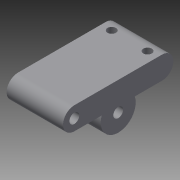
# Autodesk Inventor part: armv2
Saved by Autodesk Inventor 2015 (Build 190159000, 159)
## iProperties
Created: 2015-02-01
Part Number: armv2
Material: Generic
Document SubType Name: Modeling
Designer: Jumziey
Density: 1 g/cm^3
Appearance: Default
Author: Jumziey
Autodesk Inventor part; units mm, degrees
ref_plane "XZ Plane" through (0, 0, 0) normal (0, 1, 0) x (-1, 0, 0)
ref_plane "XY Plane" through (0, 0, 0) normal (0, 0, 1) x (1, 0, 0)
sketch "Sketch1" plane through (0, 0, 0) normal (1, 0, 0) x (0, 1, 0)
  circle A0 centre (0, 0) radius 1.75
  arc A1 (0, 4) -> (0, -4) centre (0, 0) ccw
  line L0 (0, 0) -> (15.55, 0) construction
  line L1 (15.55, -4) -> (15.55, -6) construction
  line L2 (15.55, 0) -> (31.1, 0) construction
  arc A2 (31.1, -4) -> (31.1, 4) centre (31.1, 0) ccw
  line L3 (0, 4) -> (31.1, 4)
  arc A3 (9.6814, -4) -> (21.4186, -4) centre (15.55, -6) ccw
  circle A4 centre (15.55, -6) radius 1.75
  line L4 (0, -4) -> (9.6814, -4)
  line L5 (21.4186, -4) -> (31.1, -4)
  dimension "d0" = 3.5
  dimension "d1" = 8
  dimension "d2" = 15.55
  dimension "d4" = 15.55
  dimension "d5" = 8
  dimension "d6" = 12.4
  dimension "d7" = 10
  dimension "d9" = 3.5
  dimension "d37" = 15.55
  constraints: 12 end point, 6 point on circle, 5 centre point, 5 coincident, 5 tangent, 3 horizontal
  measures "d0" diameter of A0
  measures "d1" diameter of A1
  measures "d2" distance of L0.start L0.end
  measures "d4" distance of L0.end L2.end
  measures "d5" diameter of A2
  measures "d6" diameter of A3
  measures "d7" distance from line of L1.end L3
  measures "d9" diameter of A4
  measures "d37" horizontal distance of point (0, 0) L1.end
extrude "Extrusion1" add sketch "Sketch1" along normal blind 7.3
sketch "Sketch2" plane through (7.3, 0, 0) normal (1, 0, 0) x (0, 0, -1)
  line L0 (0, 15.55) -> (6, 15.55) construction
  arc A0 (4, 21.4186) -> (4, 9.6814) centre (6, 15.55) ccw
  arc A1 (-4, 0) -> (4, 0) centre (0, 0) ccw construction
  line L1 (4, 0) -> (4, 9.6814) construction
  arc A2 (4, 31.1) -> (-4, 31.1) centre (0, 31.1) ccw construction
  line L2 (4, 21.4186) -> (4, 31.1) construction
  circle A3 centre (0, 0) radius 1.75
  arc A4 (-4, 0) -> (4, 0) centre (0, 0) ccw
  arc A5 (4, 31.1) -> (-4, 31.1) centre (0, 31.1) ccw
  line L3 (-4, 31.1) -> (-4, 0)
  line L4 (4, 0) -> (4, 9.6814)
  line L5 (-4, 31.1) -> (-4, 0) projected
  line L6 (4, 21.4186) -> (4, 31.1)
  dimension "d12" = 15.55
  dimension "d13" = 6
  dimension "d14" = 12.4
  constraints: 12 end point, 6 point on circle, 4 centre point, 4 coincident, 3 tangent, 1 parallel, 1 point on line, 1 vertical
  measures "d12" distance of point (0, 0) L0.start
  measures "d13" distance of L0.start L0.end
  measures "d14" diameter of A0
extrude "Extrusion2" add sketch "Sketch2" along normal blind 5.4
ref_plane "Work Plane1" through (12.7, 0, 0) normal (1, 0, 0) x (0, 1, 0)
sketch "Sketch3" plane through (12.7, 0, 0) normal (1, 0, 0) x (0, 1, 0)
  circle A0 centre (0, 0) radius 1.75
  arc A1 (0, 4) -> (0, -4) centre (0, 0) ccw
  line L0 (0, 0) -> (15.55, 0) construction
  line L1 (15.55, -4) -> (15.55, -6) construction
  line L2 (15.55, 0) -> (31.1, 0) construction
  arc A2 (31.1, -4) -> (31.1, 4) centre (31.1, 0) ccw
  line L3 (0, 4) -> (31.1, 4)
  arc A3 (9.6814, -4) -> (21.4186, -4) centre (15.55, -6) ccw
  circle A4 centre (15.55, -6) radius 1.75
  line L4 (0, -4) -> (9.6814, -4)
  line L5 (21.4186, -4) -> (31.1, -4)
  dimension "d18" = 3.5
  dimension "d19" = 8
  dimension "d20" = 15.55
  dimension "d21" = 15.55
  dimension "d22" = 8
  dimension "d23" = 12.4
  dimension "d24" = 10
  dimension "d26" = 3.5
  dimension "d38" = 15.55
  constraints: 12 end point, 6 point on circle, 5 centre point, 5 coincident, 5 tangent, 3 horizontal
  measures "d18" diameter of A0
  measures "d19" diameter of A1
  measures "d20" distance of L0.start L0.end
  measures "d21" distance of L0.end L2.end
  measures "d22" diameter of A2
  measures "d23" diameter of A3
  measures "d24" distance from line of L1.end L3
  measures "d26" diameter of A4
  measures "d38" horizontal distance of point (0, 0) L1.end
extrude "Extrusion3" add sketch "Sketch3" along normal blind 7.3
sketch "Sketch4" plane through (0, 0, 4) normal (0, 0, 1) x (1, 0, 0)
  circle A0 centre (3.65, 29.6) radius 1.5
  circle A1 centre (16.35, 29.6) radius 1.5
  line L0 (0, 31.1) -> (0, 0) projected
  line L1 (0, 31.1) -> (20, 31.1) projected
  line L2 (20, 31.1) -> (20, 0) projected
  dimension "d29" = 3
  dimension "d30" = 3
  dimension "d31" = 3.65
  dimension "d32" = 3.65
  constraints: 2 centre point, 2 tangent
  measures "d29" diameter of A0
  measures "d30" diameter of A1
  measures "d31" distance from line of A0.centre L0
  measures "d32" distance from line of L2 A1.centre
extrude "Extrusion5" cut sketch "Sketch4" against normal blind 8
body "Solid1"
